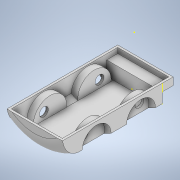
# Autodesk Inventor part: Karosserie
Saved by Autodesk Inventor 2021 (Build 250183000, 183)
## iProperties
Created: 2021-01-08
Part Number: Karosserie
Material: Generisch
Document SubType Name: Modeling
Designer: Jaro Machnow
Density: 1 g/cm^3
Appearance: Vorgabe
Author: Jaro Machnow
Autodesk Inventor part; units mm, degrees
ref_plane "YZ Plane" through (0, 0, 0) normal (1, 0, 0) x (0, 1, 0)
ref_plane "XZ Plane" through (0, 0, 0) normal (0, 1, 0) x (-1, 0, 0)
ref_plane "XY Plane" through (0, 0, 0) normal (0, 0, 1) x (1, 0, 0)
sketch "Skizze1" plane through (0, 0, 0) normal (0, 1, 0) x (-1, 0, 0)
  line L0 (125, 250) -> (-125, 250)
  line L1 (-125, 250) -> (-125, -250)
  line L2 (-125, -250) -> (125, -250)
  line L3 (125, -250) -> (125, 250)
  line L4 (0, 250) -> (0, -250) construction
  line L5 (125, 0) -> (-125, 0) construction
  point P0 (0, 0)
  dimension "Breite" = 250
  dimension "Länge" = 500
  constraints: 12 end point, 6 midpoint, 2 parallel, 1 horizontal, 1 perpendicular
  measures "Breite" distance of L2.end L1.end
  measures "Länge" distance of L1.end L0.end
extrude "Extrusion1" add sketch "Skizze1" along normal blind 80
sketch "Skizze2" plane through (0, 80, 0) normal (0, 1, 0) x (1, 0, 0)
  line L0 (-125, 250) -> (-125, -250) projected
  line L1 (125, -250) -> (125, 250) projected
  line L2 (-125, -62.8733) -> (125, -62.8733)
  line L3 (125, -62.8733) -> (125, 147.1267)
  line L4 (125, 147.1267) -> (-125, 147.1267)
  line L5 (-125, 147.1267) -> (-125, -62.8733)
  point P0 (0, 0)
  dimension "Dach_Unten_Länge" = 210
  constraints: 8 end point, 2 parallel, 2 point on line, 1 horizontal, 1 perpendicular
  measures "Dach_Unten_Länge" distance between parallel lines of L4 L2
ref_plane "Arbeitsebene1" through (0, 145, 0) normal (0, 1, 0) x (1, 0, 0)
sketch "Skizze3" plane through (0, 145, 0) normal (0, 1, 0) x (1, 0, 0)
  line L0 (-125, 250) -> (-125, -250) projected
  line L1 (125, -250) -> (125, 250) projected
  line L2 (-76.2213, -4.955) -> (76.2213, -4.955)
  line L3 (76.2213, -4.955) -> (76.2213, 113.1315)
  line L4 (76.2213, 113.1315) -> (-76.2213, 113.1315)
  line L5 (-76.2213, 113.1315) -> (-76.2213, -4.955)
  line L6 (0, -4.955) -> (0, 113.1315) construction
  point P0 (0, 0)
  constraints: 10 end point, 2 midpoint, 2 parallel, 1 horizontal, 1 perpendicular, 1 point on line
sketch "Skizze4" plane through (0, 0, 0) normal (0, 0, 1) x (1, 0, 0)
  line L0 (125, 0) -> (125, 80) projected
  arc A0 (-125, 0) -> (125, 0) centre (0, 216.5064) ccw
  line L1 (-125, 0) -> (125, 0)
  point P0 (0, 0)
  dimension "d10" = 250
  constraints: 2 end point, 2 point on circle, 1 centre point, 1 horizontal
  measures "d10" radius of A0
extrude "Extrusion2" add sketch "Skizze4" along normal mid plane 500
fillet "Rundung1" radius 80 1 edges at (0, -33.4936, 250)
ref_plane "Arbeitsebene2" through (125, 70, 238.0877) normal (1, 0, 0) x (0, 0, -1)
sketch "Skizze5" plane through (125, 70, 238.0877) normal (1, 0, 0) x (0, 0, -1)
  line L0 (488.0877, -103.4936) -> (68.0877, -103.4936) projected
  arc A0 (228.0877, -103.4936) -> (68.0877, -103.4936) centre (148.0877, -103.4936) ccw
  line L1 (68.0877, -103.4936) -> (228.0877, -103.4936)
  arc A1 (428.0877, -103.4936) -> (268.0877, -103.4936) centre (348.0877, -103.4936) ccw
  line L2 (268.0877, -103.4936) -> (428.0877, -103.4936)
  line L3 (488.0877, -103.4936) -> (438.0877, -103.4936)
  line L4 (438.0877, -103.4936) -> (438.0877, -23.4936)
  line L5 (438.0877, -23.4936) -> (488.0877, -23.4936)
  line L6 (488.0877, -23.4936) -> (488.0877, -103.4936)
  point P0 (238.0877, -70)
  dimension "d16" = 80
  dimension "d17" = 160
  dimension "d18" = 80
  dimension "d19" = 160
  dimension "Hinten_Freier_Bereich_Tiefe" = 50
  dimension "Hinten_Freie_Bereich_Hoehe" = 80
  dimension "d35" = 40
  constraints: 12 end point, 4 point on circle, 3 horizontal, 2 centre point, 2 parallel, 2 point on line, 1 perpendicular
  measures "d16" radius of A0
  measures "d17" distance of L1.end L0.end
  measures "d18" radius of A1
  measures "d19" distance of L2.end L2.start
  measures "Hinten_Freier_Bereich_Tiefe" distance of L4.end L5.end
  measures "Hinten_Freie_Bereich_Hoehe" distance of L3.end L4.end
  measures "d35" distance of L1.end L2.start
extrude "Extrusion3" cut sketch "Skizze5" against normal up to next contours L0 L4 L5 L6
ref_plane "Arbeitsebene3" through (125, 70, 238.0877) normal (1, 0, 0) x (0, 1, 0)
sketch "Skizze10" plane through (125, 70, 238.0877) normal (1, 0, 0) x (0, 1, 0)
  line L0 (-70, -68.0877) -> (-70, -438.0877) projected
  line L1 (-70, -438.0877) -> (-70, -68.0877) projected
  circle A0 centre (-70, -143.0877) radius 65
  circle A1 centre (-70, -343.0877) radius 65
  point P0 (-70, -238.0877)
  dimension "d43" = 130
  dimension "d44" = 130
  dimension "d45" = 200
  dimension "d48" = 75
  constraints: 2 centre point, 1 point on line
  measures "d43" diameter of A0
  measures "d44" diameter of A1
  measures "d45" distance of A1.centre A0.centre
  measures "d48" distance of L0.start A0.centre
extrude "Extrusion7" cut sketch "Skizze10" against normal blind 30
mirror "Spiegeln2" about plane through (0, 0, 0) normal (1, 0, 0) of "Extrusion7"
shell "Wandung2" thickness 10 removed faces 1 at (33.7738, 80, -83.3333)
ref_plane "Arbeitsebene6" through (95, -14.7403, 158.3066) normal (1, 0, 0) x (0, 1, 0)
ref_plane "Arbeitsebene5" through (0, 0, 0) normal (1, 0, 0) x (0, 1, 0)
sketch "Skizze11" plane through (95, -14.7403, 158.3066) normal (1, 0, 0) x (0, 1, 0)
  circle A0 centre (40, -35) radius 20
  line L0 (0, -126.6132) -> (0, 0) projected
  circle A1 centre (40, -286.2148) radius 20
  point P0 (14.7403, -158.3066)
  dimension "d50" = 40
  dimension "d51" = 40
  dimension "d52" = 40
  dimension "d57" = 35
  constraints: 2 centre point, 1 vertical alignment
  measures "d50" diameter of A0
  measures "d51" distance from line of A0.centre L0
  measures "d52" diameter of A1
  measures "d57" vertical distance of L0.end A0.centre
extrude "Extrusion8" cut sketch "Skizze11" against normal blind 1000
sketch "Skizze12" plane through (0, 216.5064, -190) normal (0, 0, 1) x (1, 0, 0)
  point P0 (0, -216.5064)
sketch "Skizze13" plane through (0, 216.5064, -190) normal (0, 0, 1) x (1, 0, 0)
  line L0 (-85, -141.5064) -> (-85, -224.4438) projected
  line L1 (-85, -224.4438) -> (85, -224.4438)
  arc A0 (-115, -210.6537) -> (115, -210.6537) centre (0, 0) ccw projected
  point P0 (0, -216.5064)
  constraints: 2 end point, 1 horizontal, 1 point on circle
extrude "Extrusion9" add sketch "Skizze13" along normal up to next
sketch "Skizze14" plane through (0, 216.5064, -200) normal (0, 0, -1) x (-1, 0, 0)
  line L0 (-125, -170) -> (-125, -136.5064) projected
  arc A0 (-125, -216.5064) -> (125, -216.5064) centre (0, 0) ccw projected
  line L1 (0, -250) -> (0, -173.3973)
  point P0 (0, -216.5064)
  constraints: 2 end point, 1 point on circle, 1 vertical
equation "\"Breite\" = 0.5 * Länge"
